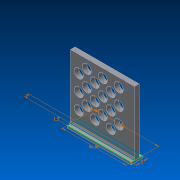
# Autodesk Inventor part: vent test circle
Saved by Autodesk Inventor 2015 (Build 190159000, 159)
## iProperties
Created: 2017-03-16
Part Number: vent test circle
Material: Generic
Document SubType Name: Modeling
Designer: ZigZagJoe
Density: 1 g/cm^3
Appearance: Default
Author: ZigZagJoe
Autodesk Inventor part; units mm, degrees
ref_plane "YZ Plane" through (0, 0, 0) normal (1, 0, 0) x (0, 1, 0)
ref_plane "XZ Plane" through (0, 0, 0) normal (0, 1, 0) x (-1, 0, 0)
ref_plane "XY Plane" through (0, 0, 0) normal (0, 0, 1) x (1, 0, 0)
sketch "Sketch1" plane through (0, 0, 0) normal (0, 0, 1) x (1, 0, 0)
  line L0 (-19.4684, -0.3877) -> (8.5316, -0.3877)
  line L1 (8.5316, -0.3877) -> (8.5316, -5.3877)
  line L2 (8.5316, -5.3877) -> (-19.4684, -5.3877)
  line L3 (-19.4684, -5.3877) -> (-19.4684, -0.3877)
  line L4 (-19.4684, -1.8877) -> (8.5316, -1.8877)
  line L5 (8.5316, -1.8877) -> (8.5316, -3.8877)
  line L6 (8.5316, -3.8877) -> (-19.4684, -3.8877)
  line L7 (-19.4684, -3.8877) -> (-19.4684, -1.8877)
  point P0 (0, 0)
  dimension "d0" = 28
  dimension "d1" = 5
  dimension "d4" = 2
  dimension "d5" = 28
  dimension "d7" = 1.5
  dimension "d56" = 0
  constraints: 16 end point, 4 parallel, 2 horizontal, 2 perpendicular
  measures "d0" distance of L1.end L2.end
  measures "d1" distance of L0.end L1.end
  measures "d4" distance of L6.end L4.start
  measures "d5" distance of L4.start L4.end
  measures "d7" distance between parallel lines of L2 L6
  measures "d56" distance between parallel lines of L3 L7
extrude "Extrusion1" add sketch "Sketch1" along normal blind 28 contours L4 L1 L6 L3
extrude "Extrusion2" add sketch "Sketch1" against normal blind 1
fillet "Fillet1" radius 1 2 edges at (-5.4684, -3.8877, 0) (-5.4684, -1.8877, 0)
sketch "Sketch2" plane through (-19.4684, -3.8877, 28) normal (0, -1, 0) x (1, 0, 0)
  line L0 (27, -1) -> (1, -1)
  line L1 (1, -1) -> (1, -17)
  line L2 (1, -17) -> (27, -17)
  line L3 (27, -17) -> (27, -1)
  line L4 (0, 0) -> (28, 0) projected
  line L5 (2.3536, -1) -> (7.3536, -1) construction
  line L6 (8.0711, -1) -> (5.2426, -3.8284)
  line L7 (5.2426, -3.8284) -> (2.4142, -1)
  line L8 (1, -2.4142) -> (3.8284, -5.2426)
  line L9 (3.8284, -5.2426) -> (1, -8.0711)
  line L10 (1, -8.0711) -> (2.4142, -9.4853)
  line L11 (2.4142, -9.4853) -> (5.2426, -6.6569)
  line L12 (5.2426, -6.6569) -> (8.0711, -9.4853)
  line L13 (8.0711, -9.4853) -> (9.4853, -8.0711)
  line L14 (9.4853, -8.0711) -> (6.6569, -5.2426)
  line L15 (6.6569, -5.2426) -> (9.4853, -2.4142)
  line L16 (9.4853, -2.4142) -> (8.0711, -1)
  line L17 (2.4142, -1) -> (1, -2.4142)
  line L18 (9.4853, -2.4142) -> (9.4853, -8.0711)
  line L19 (8.0711, -9.4853) -> (2.4142, -9.4853)
  line L20 (1, -8.0711) -> (1, -2.4142)
  line L21 (2.4142, -1) -> (8.0711, -1)
  line L22 (28, -27) -> (28, 0) projected
  line L23 (0, -27) -> (0, 0) projected
  point P0 (19.4684, -28)
  dimension "d28" = 4
  dimension "d29" = 2
  dimension "d30" = 4
  dimension "d31" = 2
  dimension "d32" = 4
  dimension "d39" = 8.4853
  dimension "d40" = 1
  dimension "d41" = 1
  dimension "d42" = 1
  constraints: 42 end point, 12 point on line, 7 perpendicular, 4 parallel, 2 horizontal, 1 collinear
  measures "d28" distance of L11.end L12.end
  measures "d29" distance of L12.end L13.end
  measures "d30" distance of L14.end L15.end
  measures "d31" distance between parallel lines of L11 L9
  measures "d32" distance of L8.start L8.end
  measures "d39" horizontal distance of L13.end L8.start
  measures "d40" distance between parallel lines of L22 L3
  measures "d41" distance between parallel lines of L23 L20
  measures "d42" distance between parallel lines of L4 L0
extrude "Extrusion3" [suppressed]
pattern_linear "Rectangular Pattern1" [suppressed]
sketch "Sketch3" plane through (-19.4684, -3.8877, 28) normal (0, -1, 0) x (1, 0, 0)
  line L0 (3, -3) -> (3, -21) construction
  line L1 (2, -3) -> (2, -21)
  line L2 (4, -21) -> (4, -3)
  arc A0 (4, -3) -> (2, -3) centre (3, -3) ccw
  arc A1 (2, -21) -> (4, -21) centre (3, -21) ccw
  line L3 (0, 0) -> (28, 0) projected
  line L4 (0, -27) -> (0, 0) projected
  point P0 (19.4684, -28)
  point P1 (3, -12)
  dimension "d43" = 2
  dimension "d44" = 3
  dimension "d45" = 18
  dimension "d48" = 3
  constraints: 8 end point, 4 point on circle, 4 tangent, 2 centre point, 1 midpoint, 1 parallel, 1 vertical
  measures "d43" diameter of A1
  measures "d44" distance from line of L0.start L3
  measures "d45" distance of L0.start L0.end
  measures "d48" distance from line of L4 L0.start
extrude "Extrusion4" [suppressed]
pattern_linear "Rectangular Pattern2" [suppressed]
fillet "Fillet2" [suppressed]
sketch "Sketch4" plane through (-19.4684, -3.8877, 28) normal (0, -1, 0) x (1, 0, 0)
  line L0 (0, -27) -> (0, 0) projected
  circle A0 centre (3.5936, -7.288) radius 2
  circle A1 centre (7.0936, -3.788) radius 2
  point P0 (19.4684, -28)
  dimension "d80" = 4
  dimension "d81" = 4
  dimension "d82" = 3.5
  dimension "d83" = 3.5
  constraints: 2 centre point
  measures "d80" diameter of A0
  measures "d81" diameter of A1
  measures "d82" horizontal distance of A1.centre A0.centre
  measures "d83" horizontal distance of A1.centre A0.centre
extrude "Extrusion5" cut sketch "Sketch4" against normal blind 10
pattern_linear "Rectangular Pattern3" count 3 spacing 7 along (1, 0, 0) count 3 spacing 7 along (0, 0, -1) of "Extrusion5"
equation "\"d0\" = d5"
equation "\"d28\" = d32"
equation "\"d29\" = d31"
equation "\"d30\" = d32"
equation "\"d80\" = d81"
equation "\"d83\" = d82"
body "Solid1"
